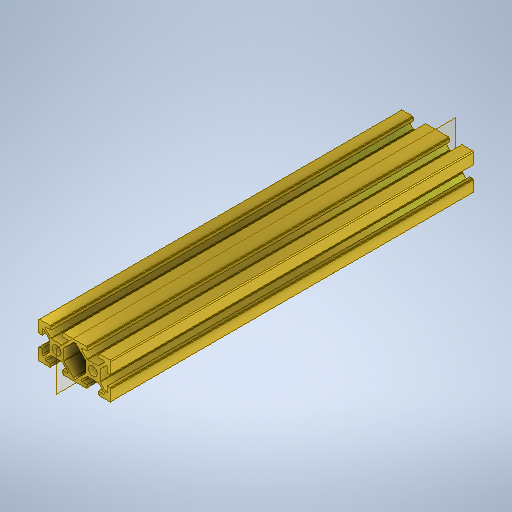
# Autodesk Inventor part: Perfil 20×40 6 rasgos_AST02004006
Saved by Autodesk Inventor 2025.2 (Build 292293000, 293)
## iProperties
Created: 2025-04-02
Part Number: Perfil 20×40 6 rasgos_AST02004006
Material: Ouro
Document SubType Name: Modeling
Designer: Gustavo Sousa
Density: 19.3 g/cm^3
Appearance: Metal quente 2400F
Author: Gustavo Sousa
Autodesk Inventor part; units mm, degrees
ref_plane "YZ Plane" through (0, 0, 0) normal (1, 0, 0) x (0, 1, 0)
ref_plane "XZ Plane" through (0, 0, 0) normal (0, 1, 0) x (-1, 0, 0)
ref_plane "XY Plane" through (0, 0, 0) normal (0, 0, 1) x (1, 0, 0)
sketch "Esboço1" plane through (0, 0, 0) normal (0, 0, 1) x (1, 0, 0)
  line L0 (-20, 10) -> (20, 10) construction
  line L1 (-3.1, 4) -> (3.1, 4) construction
  circle A0 centre (0, 0) radius 2.5 construction
  line L2 (-10, 10) -> (10, 10) construction
  line L3 (0, 0) -> (-10, 10) construction
  line L4 (3.1, 10) -> (-3.1, 10) construction
  line L5 (-10, 10) -> (-3.1, 10) construction
  line L6 (-3.1, 10) -> (-3.1, 8) construction
  line L7 (-3.1, 8) -> (-7.1, 8) construction
  line L8 (-7.1, 8) -> (-3.1, 4) construction
  line L9 (-3.1, 4) -> (0, 4) construction
  line L10 (-1.7678, 1.7678) -> (0, 0) construction
  line L11 (-1.7678, 1.7678) -> (-10, 10) construction
  line L12 (-3.1, 10) -> (-3.6, 10) construction
  line L13 (-3.6, 10) -> (-3.6, 9.5)
  line L14 (-3.6, 9.5) -> (-3.1, 9.5)
  line L15 (-3.1, 9.5) -> (-3.1, 10) construction
  line L16 (-3.1, 9.5) -> (-3.1, 8)
  line L17 (-4, 3.1) -> (-4, -3.1) construction
  line L18 (-10, 10) -> (-10, -10) construction
  line L19 (-8, 7.1) -> (-4, 3.1) construction
  line L20 (-10, 3.1) -> (-10, -3.1) construction
  line L21 (-10, 10) -> (-10, 3.1) construction
  line L22 (-10, 3.1) -> (-8, 3.1) construction
  line L23 (-8, 3.1) -> (-8, 7.1) construction
  line L24 (-10, 3.1) -> (-9.5, 3.1) construction
  line L25 (-9.5, 3.1) -> (-9.5, 3.6)
  line L26 (-9.5, 3.6) -> (-10, 3.6)
  line L27 (-10, 3.6) -> (-10, 3.1) construction
  arc A1 (-9.5, 10) -> (-10, 9.5) centre (-9.5, 9.5) ccw
  line L28 (-9.5, 10) -> (-3.6, 10)
  line L29 (-10, 9.5) -> (-10, 3.6)
  line L30 (-9.5, 3.1) -> (-8, 3.1)
  line L31 (-8, 7.1) -> (-8, 3.1) construction
  arc A2 (0, 2.5) -> (-2.5, 0) centre (0, 0) ccw
  line L32 (-2.5, 0) -> (-4, 0)
  arc A3 (-5.8929, 8) -> (-6.2464, 7.1464) centre (-5.8929, 7.5) ccw
  arc A4 (-3.2464, 4.1464) -> (-2.8929, 4) centre (-2.8929, 4.5) ccw
  line L33 (-5.8929, 8) -> (-3.1, 8)
  line L34 (-6.2464, 7.1464) -> (-3.2464, 4.1464)
  line L35 (-2.8929, 4) -> (0, 4)
  arc A5 (-7.1464, 6.2464) -> (-8, 5.8929) centre (-7.5, 5.8929) ccw
  arc A6 (-4, 2.8929) -> (-4.1464, 3.2464) centre (-4.5, 2.8929) ccw
  line L36 (-8, 5.8929) -> (-8, 3.1)
  line L37 (-7.1464, 6.2464) -> (-4.1464, 3.2464)
  line L38 (-4, 2.8929) -> (-4, 0)
  arc A7 (2.5, 0) -> (0, 2.5) centre (0, 0) ccw
  line L39 (0, 0) -> (10, 10) construction
  line L40 (10, 10) -> (3.1, 10) construction
  line L41 (3.1, 4) -> (7.1, 8) construction
  line L42 (3.1, 10) -> (3.1, 8) construction
  line L43 (3.1, 8) -> (7.1, 8) construction
  line L44 (3.1, 10) -> (3.6, 10) construction
  line L45 (3.6, 10) -> (3.6, 9.5)
  line L46 (3.6, 9.5) -> (3.1, 9.5)
  line L47 (3.1, 9.5) -> (3.1, 10) construction
  line L48 (3.6, 10) -> (10, 10)
  line L49 (3.1, 9.5) -> (3.1, 8)
  arc A8 (2.8929, 4) -> (3.2464, 4.1464) centre (2.8929, 4.5) ccw
  arc A9 (6.2464, 7.1464) -> (5.8929, 8) centre (5.8929, 7.5) ccw
  line L50 (3.1, 8) -> (5.8929, 8)
  line L51 (6.2464, 7.1464) -> (3.2464, 4.1464)
  line L52 (2.8929, 4) -> (0, 4)
  line L53 (4, -3.1) -> (4, 3.1) construction
  line L54 (4, 3.1) -> (8.9, 8) construction
  line L55 (2.5, 0) -> (4, 0) construction
  arc A10 (4.1464, 3.2464) -> (4, 2.8929) centre (4.5, 2.8929) ccw
  line L56 (4, 2.8929) -> (4, 0)
  line L57 (4.1464, 3.2464) -> (8.9, 8) construction
  line L58 (10, 10) -> (10, 9) construction
  arc A11 (10, 9) -> (9.7687, 8.8687) centre (10.1223, 8.5152) ccw
  line L59 (9.7687, 8.8687) -> (4.1464, 3.2464)
  line L60 (2.5, 0) -> (4, 0)
  line L61 (10, 10) -> (10, 9)
  point P0 (0, 10)
  point P1 (0, 10)
  point P2 (0, 10)
  point P3 (-10, 0)
  point P4 (-10, 0)
  point P5 (-1.7678, 1.7678)
  point P6 (1.7678, 1.7678)
  point P7 (3.1, 9)
  dimension "d0" = 40
  dimension "d1" = 6.2
  dimension "d3" = 5
  dimension "d6" = 10
  dimension "d7" = 6
  dimension "d8" = 20
  dimension "d11" = 2
  dimension "d15" = 0.5
  dimension "d18" = 6
  dimension "d19" = 0.5
  dimension "d21" = 4
  constraints: 124 end point, 31 point on circle, 20 point on line, 19 tangent, 14 equal length, 13 collinear, 12 centre point, 12 horizontal, 10 parallel, 9 equal radius, 9 midpoint, 8 vertical, 7 coincident, 5 horizontal alignment, 4 perpendicular, 2 vertical alignment
  measures "d0" distance of L0.start L0.end
  measures "d1" distance of L1.start L1.end
  measures "d3" diameter of A0
  measures "d6" distance from line of L0 point (0, 0)
  measures "d7" distance between parallel lines of L0 L1
  measures "d8" distance of L2.start L2.end
  measures "d11" distance between parallel lines of L5 L7
  measures "d15" distance of L13.end L12.end
  measures "d18" distance between parallel lines of L18 L17
  measures "d19" radius of A1
  measures "d21" distance from line of point (0, 0) L53
extrude "Extrusão1" add sketch "Esboço1" along normal mid plane 200
mirror "Espelhar3" about plane through (0, 0, 0) normal (0, 1, 0) of "Extrusão1"
mirror "Espelhar4" about plane through (10, 9, 0) normal (1, 0, 0) of "Extrusão1", "Espelhar3"
fillet "Arredondamento1" radius 1 1 edges at (10, 9, 0)
fillet "Arredondamento2" radius 1 1 edges at (10, -9, 0)
ref_plane "Plano de trabalho1" through (10, 3.6, -100) normal (1, 0, 0) x (0, 0, -1)
